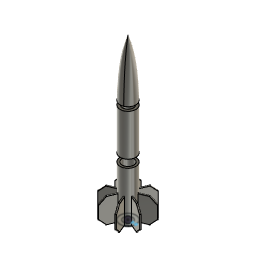
RTA1 Main v4 (Autodesk Fusion 360 design; units mm, degrees)
Autodesk Fusion 360 part; units mm, degrees
note: some values were not read from the file. Set by a fixed rule: which face or edge a step refers to.
sketch "Sketch1" plane through (0, 0, 0) normal (0, 0, 1) x (1, 0, 0)
  line L0 (0, 2.4915) -> (0, 2.4925)
  line L1 (0, 2.4925) -> (-0.0064, 2.492) construction
  line L2 (-0.0064, 2.492) -> (0, 2.4915) construction
  circle A0 centre (0, 0) radius 13.4937
  arc A1 (-2.75, 19.81) -> (-19.81, 2.75) centre (0, 0) ccw
  arc A2 (-19.81, -2.75) -> (-2.75, -19.81) centre (0, 0) ccw
  arc A3 (2.75, -19.81) -> (19.81, -2.75) centre (0, 0) ccw
  arc A4 (19.81, 2.75) -> (2.75, 19.81) centre (0, 0) ccw
  circle A5 centre (0, 0) radius 20
  line L3 (-19.81, -2.75) -> (-13.2106, -2.75)
  line L4 (-19.81, 2.75) -> (-13.2106, 2.75)
  line L5 (-2.75, -19.81) -> (-2.75, -13.2106)
  line L6 (2.75, -19.81) -> (2.75, -13.2106)
  line L7 (19.81, -2.75) -> (13.2106, -2.75)
  line L8 (19.81, 2.75) -> (13.2106, 2.75)
  line L9 (2.75, 19.81) -> (2.75, 13.2106)
  line L10 (-2.75, 19.81) -> (-2.75, 13.2106)
  dimension "d6" = 40
  dimension "d7" = 26.9875
  dimension "d83" = 40
  constraint vertical L0
  constraint coincident A2.start A1
  constraint coincident A3.start A1
  constraint coincident A2.end A1
  constraint coincident A3.end A1
  constraint coincident A4.start A1
  constraint concentric A1 A2
  constraint concentric A2 A3
  constraint concentric A3 A4
  constraint coincident A0.centre A1.centre
  constraint coincident A0 L3.end
  constraint horizontal L3
  constraint coincident A0 L4.end
  constraint parallel L3 L4
  constraint coincident A0 L5.end
  constraint perpendicular L4 L5
  constraint coincident A0 L6.end
  constraint parallel L5 L6
  constraint coincident A0 L7.end
  constraint perpendicular L6 L7
  constraint coincident A0 L8.end
  constraint parallel L7 L8
  constraint coincident A0 L9.end
  constraint perpendicular L8 L9
  constraint coincident A0 L10.end
  constraint parallel L9 L10
  measures "d6" diameter of A1
  measures "d7" diameter of A0
  measures "d83" diameter of A5
extrude "Extrude1" add sketch "Sketch1" along normal blind 127 contours A0 A5 L7 L8 | A0 A4 A5 L8 L9 | A0 A3 A5 L6 L7 | A0 A5 L9 L10 | A0 A5 L5 L6 | A0 A1 A5 L4 L10 | A0 A2 A5 L3 L5 | A0 A5 L3 L4 makes body 1
move_body "Move1" bodies 1 to x (0.707107, -0.707107, 0) y (0.707107, 0.707107, 0) z (0, 0, 1) at (0, 0, 0)
sketch "Sketch5" plane through (0, 0, 127) normal (0, 0, 1) x (-1, 0, 0)
  circle A0 centre (0, 0) radius 13.4937
  circle A1 centre (0, 0) radius 20
  circle A2 centre (0, 0) radius 20
  dimension "d105" = 40
  measures "d105" diameter of A2
extrude "Extrude8" add sketch "Sketch5" along normal blind 20 and the other way blind -15 separate body contours A0 | A1 A2 makes body 2
ref_plane "WorkPlane1" through (0, 0, 300) normal (0, 0, 1) x (1, 0, 0)
ref_plane "WorkPlane2" through (0, 0, 475) normal (0, 0, 1) x (1, 0, 0)
extrude "Extrude14" add sketch "Sketch5" along normal blind 120 and the other way blind -15 contours A0 | A1 A2 bodies 2
extrude "Extrude15" cut sketch "Sketch1" along normal blind 170 contours A0 bodies 2
sketch "Sketch9" plane through (0, 0, 0) normal (1, 0, 0) x (0, 1, 0)
  line L0 (0, 255.8937) -> (-20, 255.8937)
  spline S0 degree 5 poles (-20, 255.8937) (-19.9774, 257.0879) (-19.9266, 259.5107) (-19.8335, 263.2483) (-19.6751, 268.4392) (-19.4188, 275.2738) (-19.1015, 282.4453) (-18.7189, 289.9296) (-18.2647, 297.678) (-17.7307, 305.6153) (-17.1077, 313.6533) (-16.3855, 321.6999) (-15.5543, 329.6706) (-14.605, 337.4982) (-13.5301, 345.1449) (-12.324, 352.5964) (-10.9822, 359.8546) (-9.5021, 366.9313) (-7.8823, 373.8423) (-6.1234, 380.6006) (-4.2275, 387.215) (-2.6029, 392.3963) (-1.3246, 396.2217) (-0.4459, 398.745) (0, 400) knots 0 0 0 0 0 0 0.05 0.1 0.15 0.2 0.25 0.3 0.35 0.4 0.45 0.5 0.55 0.6 0.65 0.7 0.75 0.8 0.85 0.9 0.95 1 1 1 1 1 1
  line L1 (0, 400) -> (0, 255.8937)
  point P0 (-18.8373, 287.4604)
  point P1 (-15.4325, 330.447)
  point P2 (-9.0483, 368.7519)
  dimension "d90" = 20
  constraint horizontal L0
  constraint perpendicular L0 L1
  measures "d90" distance of L0.start L0.end
revolve "Revolve2" add sketch "Sketch9" angle 360 about axis through (0, 0, 1.75) along (0, 0, 1) separate body makes body 3
sketch "Sketch10" plane through (0, 0, 255.8937) normal (0, 0, -1) x (1, 0, 0)
  circle A0 centre (0, 0) radius 20
  circle A1 centre (0, 0) radius 13.5
  dimension "d92" = 27
  constraint concentric A0 A1
  measures "d92" diameter of A1
extrude "Extrude16" add sketch "Sketch10" along normal blind 5 contours A1 bodies 3
move_body "Move14" bodies 2 to x (1, 0, 0) y (0, 1, 0) z (0, 0, 1) at (0, 0, -5)
sketch "Sketch11" plane through (0, 0, 0) normal (0, 0, -1) x (1, 0, 0)
  circle A0 centre (0, 0) radius 13.4937
  circle A1 centre (0, 0) radius 20
  line L0 (20, -0.0306) -> (57.9413, -0.0306)
  line L1 (57.9413, -0.0306) -> (57.9413, -1.5306)
  line L2 (57.9413, -1.5306) -> (57.9413, 1.4694)
  line L3 (57.9413, 1.4694) -> (19.9459, 1.4694)
  line L4 (57.9413, -1.5306) -> (19.9413, -1.5306)
  arc A2 (19.9413, -1.5306) -> (19.9459, 1.4694) centre (0, 0) ccw
  dimension "d118" = 1.5
  dimension "d119" = 3
  dimension "d120" = 38
  constraint horizontal L0
  constraint perpendicular L0 L1
  constraint perpendicular L0 L2
  constraint perpendicular L1 L3
  constraint perpendicular L1 L4
  constraint coincident A1 L3.end
  constraint coincident A1 L4.end
  constraint coincident A1 L0.start
  measures "d118" distance of L0.end L1.end
  measures "d119" distance of L1.end L2.end
  measures "d120" distance of L1.end L4.end
extrude "Extrude17" add sketch "Sketch11" against normal blind 65 separate body contours A1 L0 L2 L3 A2 | A1 L0 L1 L2 L4 A2 makes body 4
move_body "Move15" bodies 2 to x (1, 0, 0) y (0, 1, 0) z (0, 0, 1) at (0, 0, -10)
move_body "Move16" bodies 3 to x (1, 0, 0) y (0, 1, 0) z (0, 0, 1) at (0, 0, -23.8)
move_body "Move18" bodies 3 to x (1, 0, 0) y (0, 1, 0) z (0, 0, 1) at (0, 0, 30)
move_body "Move19" bodies 2 to x (1, 0, 0) y (0, 1, 0) z (0, 0, 1) at (0, 0, 20)
extrude "Extrude18" cut 1 faces at (-3.6924, 4.3406, 175) along direction (0, 0, 1) blind 80 on bodies 2 bodies 2
chamfer "Chamfer5" distance 15 angle 45 2 edges at (57.9413, 0.0306, 65) (57.9413, 0.0306, 0) on bodies 4
fillet "Fillet8" radius 1.5 8 edges at (31.4436, -1.4694, 65) (31.4413, 1.5306, 65) (31.4436, -1.4694, 0) (31.4413, 1.5306, 0) (50.4413, 1.5306, 7.5) (50.4413, 1.5306, 57.5) (50.4413, -1.4694, 57.5) (50.4413, -1.4694, 7.5) on bodies 4
pattern_circular "C-Pattern5" count 8 over 360 about axis through (0, 0, 1.75) along (0, 0, 1) of bodies 4 makes body 5 at (21.9751, 24.1396, 37.6264) makes body 6 at (-1.5306, 32.608, 37.6264) makes body 7 at (-24.1396, 21.9751, 37.6264) makes body 8 at (-32.608, -1.5306, 37.6264) makes body 9 at (-21.9751, -24.1396, 27.3736) makes body 10 at (1.5306, -32.608, 37.6264) makes body 11 at (24.1396, -21.9751, 37.6264)
move_face "OffsetFaces1" offset -1.98 9 faces at (9.7566, -9.3215, 84.6667) (8.6327, -10.371, 84.6667) (-4.48, -12.7284, 84.6667) (-7.9036, -10.9368, 84.6667) (-12.7284, -4.48, 84.6667) (-10.9368, 7.9036, 84.6667) (-6.8427, 11.6301, 84.6667) (10.9368, 7.9036, 42.3333) (11.6301, 6.8427, 84.6667) on bodies 1
move_face "OffsetFaces2" offset 1.948 9 faces at (12.1154, -9.6257, 84.6667) (9.8994, -11.8928, 84.6667) (-2.9738, -15.1853, 42.3333) (-12.5417, -9.0633, 42.3333) (-13.7003, 7.193, 84.6667) (-9.0633, 12.5417, 42.3333) (2.9738, 15.1853, 84.6667) (12.5417, 9.0633, 42.3333) (15.4557, -0.7478, 84.6667) on bodies 1
move_face "OffsetFaces3" offset -1.952 9 faces at (10.5902, -8.4139, 84.6667) (8.6532, -10.3956, 84.6667) (-3.2379, -13.1325, 84.6667) (-10.9628, -7.9223, 42.3333) (-11.6577, 6.8589, 42.3333) (-7.9223, 10.9628, 42.3333) (4.4906, 12.7585, 84.6667) (10.9628, 7.9223, 42.3333) (13.4626, 1.3058, 84.6667) on bodies 1
move_face "OffsetFaces4" offset 1 9 faces at (11.8958, -9.902, 42.3333) (9.6282, -12.1185, 42.3333) (-5.1387, -14.5998, 84.6667) (-12.5449, -9.0657, 42.3333) (-13.3401, 7.8488, 42.3333) (-9.0657, 12.5449, 42.3333) (5.1387, 14.5998, 84.6667) (12.5449, 9.0657, 42.3333) (15.4055, 1.4943, 84.6667) on bodies 1
move_face "OffsetFaces5" offset -0.5 9 faces at (11.3356, -9.0061, 84.6667) (9.2622, -11.1273, 84.6667) (-3.4658, -14.0568, 84.6667) (-11.7344, -8.4799, 42.3333) (-12.4782, 7.3417, 42.3333) (-8.4799, 11.7344, 42.3333) (2.7824, 14.2079, 84.6667) (11.7344, 8.4799, 42.3333) (13.6565, -4.8067, 84.6667) on bodies 1
move_face "OffsetFaces6" offset 0.478 9 faces at (11.7271, -9.3171, 84.6667) (9.5821, -11.5116, 84.6667) (-3.5855, -14.5423, 84.6667) (-12.1396, -8.7728, 42.3333) (-12.9091, 7.5952, 42.3333) (-8.7728, 12.1396, 42.3333) (4.9727, 14.1282, 84.6667) (12.1396, 8.7728, 42.3333) (14.5423, 3.5855, 84.6667) on bodies 1
move_face "OffsetFaces7" offset -0.05 9 faces at (11.3528, -9.0198, 84.6667) (9.2763, -11.1442, 84.6667) (-3.471, -14.0782, 84.6667) (-11.7522, -8.4928, 42.3333) (-12.4972, 7.3528, 42.3333) (-8.4928, 11.7522, 42.3333) (2.7866, 14.2295, 84.6667) (11.7522, 8.4928, 42.3333) (14.2295, -2.7866, 84.6667) on bodies 1
sketch "Sketch12" plane through (0, 0, 0) normal (0, 0, 1) x (1, 0, 0)
  circle A0 centre (0, 0) radius 11.1125
  line L0 (10.9829, 1.6925) -> (8.9829, 1.6925)
  line L1 (8.9829, 1.6925) -> (8.9829, -1.6915)
  line L2 (8.9829, -1.6915) -> (10.9829, -1.6915)
  line L3 (10.9829, -1.6915) -> (10.9829, 1.6925)
  circle A1 centre (0, 0) radius 20
  line L4 (19.9283, -1.6915) -> (21.9283, -1.6915)
  line L5 (21.9283, -1.6915) -> (21.9283, 1.6925)
  line L6 (21.9283, 1.6925) -> (19.9283, 1.6925)
  line L7 (19.9283, 1.6925) -> (19.9283, -1.6915)
  line L8 (19.9283, -1.6915) -> (10.9829, -1.6915)
  line L9 (10.9829, -1.6915) -> (10.9829, 1.6925)
  line L10 (10.9829, 1.6925) -> (19.9283, 1.6925)
  line L11 (19.9283, 1.6925) -> (19.9283, -1.6915)
  dimension "d130" = 22.225
  dimension "d131" = 2
  dimension "d132" = 3.384
  dimension "d133" = 40
  dimension "d134" = 2
  constraint coincident A0.centre A1.centre
  constraint horizontal L0
  constraint vertical L1
  constraint horizontal L2
  constraint vertical L3
  constraint coincident A0 L0.start
  constraint concentric A0 A1
  constraint horizontal L4
  constraint vertical L5
  constraint horizontal L6
  constraint vertical L7
  constraint coincident A1 L4.start
  constraint horizontal L8
  constraint vertical L9
  constraint horizontal L10
  constraint vertical L11
  measures "d130" diameter of A0
  measures "d131" distance of L0.start L0.end
  measures "d132" distance of L0.start L2.end
  measures "d133" diameter of A1
  measures "d134" distance of L4.start L4.end
extrude "Extrude19" add sketch "Sketch12" against normal blind 3.5 separate body contours L0 L1 L2 L3 L9 | A1 L4 L5 L6 makes body 12 at (10.9829, -0.5635, -1.1667) makes body 13 at (19.9566, 1.3171, -2.3333)
extrude "Extrude20" add sketch "Sketch12" along normal blind -3.5 and the other way blind 2 separate body contours A0 L7 L8 L10 L11 makes body 14
combine "Combine1" operation add target body 12 tool bodies 13 14
extrude "Extrude21" add sketch "Sketch12" along normal blind -3.5 and the other way blind 2 separate body contours A0 L3 L9 makes body 15
extrude "Extrude22" add sketch "Sketch12" along normal blind -3.5 and the other way blind 2 separate body contours A1 L7 L11 makes body 16
combine "Combine2" operation add target body 12 tool bodies 15 16
move_body "Move20" bodies 1 2 8 11 5 7 9 3 10 4 6 to x (0.92388, 0.382683, 0) y (-0.382683, 0.92388, 0) z (0, 0, 1) at (0, 0, 0)
pattern_circular "C-Pattern6" count 4 over 360 about axis through (0, 0, 1.75) along (0, 0, 1) of bodies 12 makes body 17 at (-0.5645, 13.298, -3.5) makes body 18 at (-13.298, -0.5645, -3.5) makes body 19 at (0.5645, -13.298, -3.5)
equation "d90 = ( 40 / 2 ) * 1 mm"
equation "d124 = 30.948 mm - 29 mm"
equation "d125 = -( 29 mm - 27.048 mm )"
equation "d128 = ( 0.956 / 2 ) * 1 mm"
equation "d132 = ( 1.692 * 2 ) * 1 mm"
named bodies: "Fuselg. 1", "Nose", "Fin 1", "ChuteBay", "Fin 2", "Fin 3", "Fin 4", "Fin 5", "Fin 6", "Fin 7", "Fin 8", "Clip 1", "Clip 2", "Clip 3", "Clip 4"
